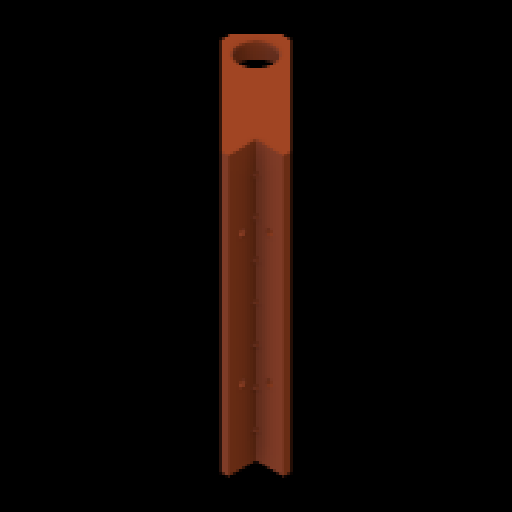
# Autodesk Inventor part: Corner Z Brace w Bearing
Saved by Autodesk Inventor 2023.2 (Build 272271000, 271)
## iProperties
Created: 2023-02-15
Part Number: Corner Z Brace w Bearing
Material: ABS Plastic
Document SubType Name: Modeling
Designer: remop
Density: 1.06 g/cm^3
Appearance: Smooth - Light Orange
Author: remop
Autodesk Inventor part; units mm, degrees
ref_plane "YZ Plane" through (0, 0, 0) normal (1, 0, 0) x (0, 1, 0)
ref_plane "XZ Plane" through (0, 0, 0) normal (0, 1, 0) x (-1, 0, 0)
ref_plane "XY Plane" through (0, 0, 0) normal (0, 0, 1) x (1, 0, 0)
sketch "Sketch1" plane through (0, 0, 0) normal (0, 1, 0) x (-1, 0, 0)
  line L0 (0, 0) -> (0, 15)
  line L1 (0, 15) -> (14.1421, 15)
  line L2 (14.1421, 15) -> (14.1421, 0)
  line L3 (14.1421, 0) -> (0, -14.1421)
  line L4 (0, -14.1421) -> (-15, -14.1421)
  line L5 (-15, -14.1421) -> (-15, 0)
  line L6 (-15, 0) -> (0, 0)
  dimension "d0" = 15
  dimension "d1" = 10
  constraints: 14 end point, 7 perpendicular, 1 parallel, 1 point on line, 1 vertical
  measures "d0" distance of L0.start L0.end
  measures "d1" distance from line of L0.start L3
extrude "Extrusion1" add sketch "Sketch1" along normal blind 151
chamfer "Chamfer1" distance 10 angle 45 2 edges at (-14.1421, 75.5, 15) (15, 75.5, -14.1421)
sketch "Sketch2" plane through (0, 151, 0) normal (0, 1, 0) x (1, 0, 0)
  line L0 (5, 14.1421) -> (15, 4.1421) projected
  line L1 (5, 14.1421) -> (0, 14.1421) projected
  line L2 (0, 14.1421) -> (-14.1421, 0) projected
  line L3 (-14.1421, 0) -> (-14.1421, -5) projected
  line L4 (-4.1421, -15) -> (-14.1421, -5) projected
  line L5 (-4.1421, -15) -> (0, -15) projected
  line L6 (0, -15) -> (0, 0) projected
  line L7 (0, 0) -> (15, 0) projected
  line L8 (15, 0) -> (15, 4.1421) projected
  circle A0 centre (-39.9264, 39.9264) radius 11.15
  line L9 (5, 14.1421) -> (-37.4264, 56.5685)
  line L10 (-37.4264, 56.5685) -> (-42.4264, 56.5685)
  line L11 (-42.4264, 56.5685) -> (-56.5685, 42.4264)
  line L12 (-56.5685, 42.4264) -> (-56.5685, 37.4264)
  line L13 (-56.5685, 37.4264) -> (-14.1421, -5)
  line L14 (-4.1421, -15) -> (-14.1421, -5) projected
  line L15 (5, 14.1421) -> (15, 4.1421) projected
  line L16 (-14.1421, 0) -> (-14.1421, -5) projected
  dimension "d7" = 22.3
  dimension "d8" = 60
  dimension "d9" = 27.0711
  dimension "d10" = 13.5355
  dimension "d11" = 13.5355
  constraints: 10 end point, 3 equal length, 2 collinear, 1 centre point, 1 horizontal, 1 perpendicular
  measures "d7" diameter of A0
  measures "d8" distance of L12.end L3.end
  measures "d9" distance between parallel lines of L9 L13
  measures "d10" distance from line of L13 A0.centre
  measures "d11" distance from line of L11 A0.centre
extrude "Extrusion2" add sketch "Sketch2" against normal blind 10 contours L1 L2 L3 L13 L12 L11 L10 L9
sketch "Sketch3" plane through (0, 151, 0) normal (0, 1, 0) x (1, 0, 0)
  circle A0 centre (-39.9264, 39.9264) radius 11.15 projected
  circle A1 centre (-39.9264, 39.9264) radius 9.15
  point P0 (0, 0)
  dimension "d14" = 2
  constraints: 1 centre point, 1 coincident
  measures "d14" radial gap between concentric circles of A0 A1
extrude "Extrusion3" add sketch "Sketch3" against normal blind 2
sketch "Sketch4" plane through (-14.1421, 0, 0) normal (-1, 0, 0) x (0, 0, 1)
  line L0 (5, 141) -> (0, 141) projected
  line L1 (0, 0) -> (0, 141) projected
  line L2 (0, 0) -> (5, 0) projected
  line L3 (5, 141) -> (5, 0) projected
  line L4 (-37.4264, 151) -> (15, 151) projected
  line L5 (-37.4264, 151) -> (-37.4264, 141) projected
  line L6 (5, 141) -> (-37.4264, 141) projected
  line L7 (5, 141) -> (5, 0) projected
  line L8 (5, 0) -> (15, 0) projected
  line L9 (15, 0) -> (15, 151) projected
  point P0 (0, 0)
  point P1 (7.5, 40)
  point P2 (7.5, 111)
  dimension "d17" = 7.5
  dimension "d18" = 40
  dimension "d19" = 40
  constraints: 1 vertical alignment
  measures "d17" distance from line of L9 point (7.5, 40)
  measures "d18" distance from line of L8 point (7.5, 40)
  measures "d19" distance from line of L4 point (7.5, 111)
hole "Hole1" at (-14.1421, 40, 7.5) at (-14.1421, 111, 7.5) direction (1, 0, 0) diameter 3.6 end through all counterbore diameter 6.5 counterbore depth 10 clearance for "Hex Head Cap Screw ISO 24017" size "M3" standard "ISO"
sketch "Sketch5" plane through (5, 0, -14.1421) normal (0, 0, -1) x (-1, 0, 0)
  line L0 (5, 141) -> (0, 141) projected
  line L1 (0, 0) -> (0, 141) projected
  line L2 (0, 0) -> (5, 0) projected
  line L3 (5, 0) -> (5, 141) projected
  line L4 (-10, 151) -> (42.4264, 151) projected
  line L5 (-10, 151) -> (-10, 0) projected
  line L6 (-10, 0) -> (0, 0) projected
  line L7 (0, 0) -> (0, 141) projected
  line L8 (42.4264, 141) -> (0, 141) projected
  line L9 (42.4264, 151) -> (42.4264, 141) projected
  point P0 (-2.5, 40)
  point P1 (-2.5, 111)
  dimension "d27" = 7.5
  dimension "d28" = 40
  dimension "d29" = 40
  constraints: 1 vertical alignment
  measures "d27" distance from line of L5 point (-2.5, 40)
  measures "d28" distance from line of L6 point (-2.5, 40)
  measures "d29" distance from line of L4 point (-2.5, 111)
hole "Hole2" at (7.5, 40, -14.1421) at (7.5, 111, -14.1421) direction (0, 0, 1) diameter 3.6 end through all counterbore diameter 6.5 counterbore depth 10 clearance for "Hex Head Cap Screw ISO 24017" size "M3" standard "ISO"
sketch "Sketch6" plane through (0, 0, -14.1421) normal (-0.7071, 0, -0.7071) x (-0.7071, 0, 0.7071)
  circle A0 centre (10, -125) radius 3 projected
  circle A1 centre (10, -85) radius 3 projected
  circle A2 centre (10, -45) radius 3 projected
  circle A3 centre (10, -5) radius 3 projected
  circle A4 centre (10, 35) radius 3 projected
  circle A5 centre (10, 75) radius 3 projected
  circle A6 centre (10, 115) radius 3 projected
  circle A7 centre (10, 135) radius 3 projected
  circle A8 centre (10, 95) radius 3 projected
  circle A9 centre (10, 55) radius 3 projected
  circle A10 centre (10, 15) radius 3 projected
  circle A11 centre (10, -25) radius 3 projected
  circle A12 centre (10, -65) radius 3 projected
  circle A13 centre (10, -105) radius 3 projected
  circle A14 centre (10, -145) radius 3 projected
  line L0 (14.5, 140) -> (5.5, 140) projected
  line L1 (5.5, 140) -> (5.5, -210) projected
  line L2 (14.5, -210) -> (5.5, -210) projected
  line L3 (14.5, 140) -> (14.5, -210) projected
  circle A15 centre (10, -205) radius 3 projected
  circle A16 centre (10, -165) radius 3 projected
  circle A17 centre (10, -185) radius 3 projected
  point P0 (10, 0)
hole "Hole3" at (-7.0711, 15, -7.0711) at (-7.0711, 35, -7.0711) at (-7.0711, 55, -7.0711) at (-7.0711, 75, -7.0711) at (-7.0711, 95, -7.0711) at (-7.0711, 115, -7.0711) at (-7.0711, 135, -7.0711) direction (0.7071, 0, 0.7071) diameter 2.8 end through all
equation "\"d10\" = 0.5 * d9"
equation "\"d11\" = d10"
equation "\"d19\" = d18"
equation "\"d29\" = d28"
body "Solid1"
